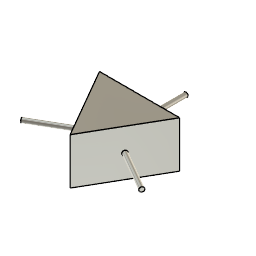
wrist_integrator (Autodesk Fusion 360 design; units mm, degrees)
Autodesk Fusion 360 part; units mm, degrees
sketch "Çizim1" plane through (0, 0, 0) normal (0, 0, 1) x (1, 0, 0)
  line L0 (-86.6025, 50) -> (0, -100)
  line L1 (0, -100) -> (86.6025, 50)
  line L2 (86.6025, 50) -> (-86.6025, 50)
  dimension "d1" = 50
  measures "d1" distance of origin L2
extrude "Ekstrüzyon1" add sketch "Çizim1" along normal blind 100 makes body 1
sketch "Çizim2" plane through (43.3013, -25, 0) normal (0.866025, -0.5, 0) x (0.5, 0.866025, 0)
  line L0 (-86.6025, 0) -> (86.6025, 0)
  line L1 (86.6025, 0) -> (86.6025, 100)
  line L2 (86.6025, 100) -> (-86.6025, 100)
  line L3 (-86.6025, 100) -> (-86.6025, 0)
  circle A0 centre (0, 50) radius 5
  dimension "d4" = 10
  measures "d4" diameter of A0
extrude "Ekstrüzyon2" add sketch "Çizim2" along normal blind 100 contours A0 bodies 1
split "Böl1" by plane through (0, -100, 0) normal (0.866025, -0.5, 0) bodies 1 makes body 2 at (100.6022, -59.0853, 54.924)
sketch "Çizim3" plane through (0, 50, 0) normal (0, 1, 0) x (-1, 0, 0)
  line L0 (-86.6025, 0) -> (86.6025, 0)
  line L1 (86.6025, 0) -> (86.6025, 100)
  line L2 (86.6025, 100) -> (-86.6025, 100)
  line L3 (-86.6025, 100) -> (-86.6025, 0)
  circle A0 centre (0, 50) radius 5
  dimension "d7" = 10
  measures "d7" diameter of A0
extrude "Ekstrüzyon3" add sketch "Çizim3" along normal blind 100 contours A0 bodies 1
sketch "Çizim4" plane through (-43.3013, -25, 0) normal (-0.866025, -0.5, 0) x (0.5, -0.866025, 0)
  line L0 (-86.6025, 0) -> (86.6025, 0)
  line L1 (86.6025, 0) -> (86.6025, 100)
  line L2 (86.6025, 100) -> (-86.6025, 100)
  line L3 (-86.6025, 100) -> (-86.6025, 0)
  circle A0 centre (0, 50) radius 5
  dimension "d10" = 10
  measures "d10" diameter of A0
extrude "Ekstrüzyon4" add sketch "Çizim4" along normal blind 100 contours A0 bodies 1
